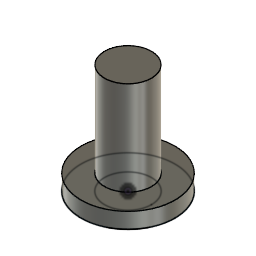
lenmount_screw (Autodesk Fusion 360 design; units mm, degrees)
part number: 2025-12-16-23-01-08-189
Autodesk Fusion 360 part; units mm, degrees
sketch "Sketch1" plane through (0, 0, 0) normal (0, 0, 1) x (1, 0, 0)
  circle A0 centre (0, 0) radius 3
  circle A1 centre (0, 0) radius 1.5
  dimension "d1" = 6
  dimension "d2" = 3
  constraint coincident A0.centre A1.centre
  constraint concentric A0 A1
  measures "d1" diameter of A0
  measures "d2" diameter of A1
extrude "Extrude1" add sketch "Sketch1" along normal blind 1
extrude "Extrude2" add sketch "Sketch1" along normal blind 7 contours A1
move_face "OffsetFaces1" [suppressed]
